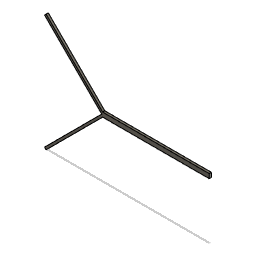
y_junction (Autodesk Fusion 360 design; units mm, degrees)
Autodesk Fusion 360 part; units mm, degrees
sketch "Sketch1" plane through (0, 0, 0) normal (0, 0, 1) x (1, 0, 0)
  line L0 (0.0707, 5.374) -> (5.374, 0.0707)
  line L1 (5.374, 0.0707) -> (5.2326, -0.0707)
  line L2 (5.2326, -0.0707) -> (-0.0707, 5.2326)
  line L3 (-0.0707, 5.2326) -> (0.0707, 5.374)
  line L4 (0, 0) -> (25, 0) construction
  line L5 (0.0707, -5.374) -> (5.374, -0.0707)
  line L6 (-0.0707, -5.2326) -> (0.0707, -5.374)
  line L7 (5.2326, 0.0707) -> (-0.0707, -5.2326)
  line L8 (5.374, -0.0707) -> (5.2326, 0.0707)
  line L9 (5.1619, 0.2) -> (15, 0.2)
  line L10 (15, 0.2) -> (15, -0.2)
  line L11 (15, -0.2) -> (5.1619, -0.2)
  line L12 (5.1619, -0.2) -> (5.1619, 0.2)
  line L13 (0, -5.3033) -> (0, 5.3033) construction
  point P0 (0, 5.3033)
  point P1 (0, -5.3033)
  point P2 (5.3033, 0)
  point P3 (5.1619, 0)
  dimension "d39" = 25
  dimension "d40" = 0.2
  dimension "d41" = 45
  dimension "d42" = 0.4
  dimension "d46" = 15
  dimension "d48" = 7.5
  constraint midpoint P0 L3
  constraint midpoint P2 L1
  constraint coincident L4.start origin
  constraint coincident P2 L4
  constraint parallel L0 L2
  constraint parallel L1 L3
  constraint perpendicular L0 L3
  constraint symmetric L0.start L4 L5.start
  constraint symmetric L0.end L4 L5.end
  constraint symmetric L1.end L4 L7.start
  constraint symmetric L2.end L4 L6.start
  constraint horizontal L9
  constraint vertical L10
  constraint horizontal L11
  constraint vertical L12
  constraint midpoint L12 P3
  constraint midpoint P1 L6
  constraint coincident P1 L13.start
  constraint coincident P0 L13.end
  constraint vertical L13
  constraint coincident L4.start L13
  constraint coincident L4 P3
  constraint coincident L2 P3
  measures "d39" distance of L4.start L4.end
  measures "d40" distance of L0 L2
  measures "d41" angle of L4 L7
  measures "d42" distance of L9.start L11.end
  measures "d46" distance of L10 L13
  measures "d48" distance of L5.start L5.end
extrude "Extrude1" add sketch "Sketch1" along normal blind 0.2
equation "d1001 = depth"
equation "channelwidth = 0.2 mm"
equation "depth = 0.2 mm"
equation "length = 15 mm"
equation "d40 = channelwidth"
equation "d41 = angle"
equation "d42 = channelwidth * 2"
equation "angle = 45 deg"
equation "d46 = length"
equation "d48 = length / 2"
equation "combinedwidth = channelwidth * 2"
